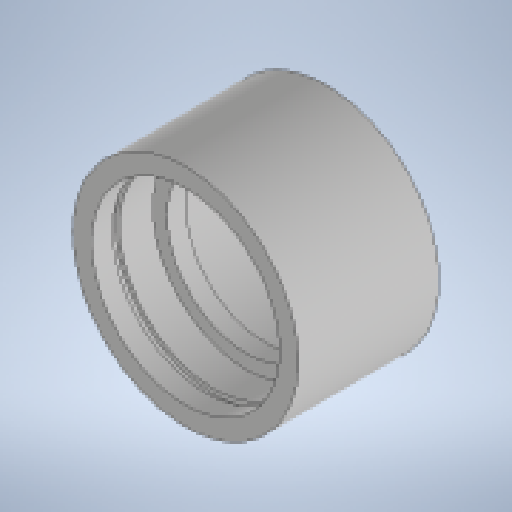
# Autodesk Inventor part: Седло для подшипника
Saved by Autodesk Inventor 2025 (Build 290162010, 162A)
## iProperties
Created: 2024-07-07
Part Number: Седло для подшипника
Material: Generic
Document SubType Name: Modeling
Designer: pokla
Density: 1 g/cm^3
Appearance: Default
Stock Number: Седло для подшипника
Author: pokla
Autodesk Inventor part; units mm, degrees
ref_plane "YZ Plane" through (0, 0, 0) normal (1, 0, 0) x (0, 1, 0)
ref_plane "XZ Plane" through (0, 0, 0) normal (0, 1, 0) x (-1, 0, 0)
ref_plane "XY Plane" through (0, 0, 0) normal (0, 0, 1) x (1, 0, 0)
sketch "Sketch6" plane through (0, 0, 0) normal (0, 0, 1) x (1, 0, 0)
  line L0 (20, 15) -> (24, 15)
  line L1 (24, 15) -> (24, -15)
  line L2 (24, -15) -> (20, -15)
  line L3 (20, -15) -> (20, -10.6)
  line L4 (17, 2) -> (20, 2)
  line L5 (20, 2) -> (20, -2) construction
  line L6 (20, -2) -> (17, -2)
  line L7 (17, -2) -> (17, 2)
  line L8 (20, -9) -> (21, -9)
  line L9 (21, -9) -> (21, -10.6)
  line L10 (21, -10.6) -> (20, -10.6)
  line L11 (20, -10.6) -> (20, -9) construction
  line L12 (20, 2) -> (20, 15)
  line L13 (20, -2) -> (20, 2) construction
  line L14 (20, -9) -> (20, -2)
  line L15 (20, -10.6) -> (20, -9) construction
  line L16 (0, 0) -> (0, 29.8024)
  point P0 (24, 0)
  point P1 (20, 0)
  point P2 (20, -9.8)
  point P3 (20.5, -9)
  dimension "d15" = 4
  dimension "d16" = 3
  dimension "d17" = 7
  dimension "d18" = 1.6
  dimension "d19" = 1
  dimension "d21" = 48
  dimension "d22" = 40
  dimension "d23" = 30
  constraints: 34 end point, 10 parallel, 4 midpoint, 3 horizontal, 3 perpendicular, 2 horizontal alignment, 1 vertical, 1 vertical alignment
  measures "d15" distance of L6.end L4.start
  measures "d16" distance of L5.end L6.end
  measures "d17" distance from line of point (20.5, -9) L6
  measures "d18" distance of L8.end L9.end
  measures "d19" distance of L9.end L3.end
  measures "d21" diameter of L1 L16
  measures "d22" diameter of L12 L16
  measures "d23" distance of L0.end L1.end
revolve "Revolution1" add sketch "Sketch6" angle 360 mid plane about axis through (0, 0, 0) along (0, 1, 0)
body "Solid2"
